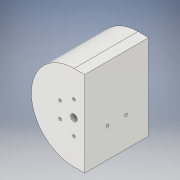
# Autodesk Inventor part: AA004
Saved by Autodesk Inventor 2017 SP1 (Build 210196100, 196)
## iProperties
Created: 2017-09-28
Part Number: AA004
Material: ABS Plastic
Document SubType Name: Modeling
Designer: Zach
Density: 1.06 g/cm^3
Appearance: CR White
Author: Zach
Autodesk Inventor part; units mm, degrees
ref_plane "YZ Plane" through (0, 0, 0) normal (1, 0, 0) x (0, 1, 0)
ref_plane "XZ Plane" through (0, 0, 0) normal (0, 1, 0) x (-1, 0, 0)
ref_plane "XY Plane" through (0, 0, 0) normal (0, 0, 1) x (1, 0, 0)
sketch "Sketch1" plane through (0, 0, 0) normal (0, 0, 1) x (1, 0, 0)
  circle A0 centre (0, 0) radius 80 construction
  line L0 (0, 80) -> (20, 80)
  line L1 (0, -80) -> (20, -80)
  line L2 (20, -80) -> (20, 80)
  arc A1 (0, 80) -> (0, -80) centre (0, 0) ccw
  circle A2 centre (0, 0) radius 6.15
  dimension "d0" = 160
  dimension "d1" = 20
  dimension "d3" = 12.3
  constraints: 6 end point, 4 point on circle, 3 centre point, 3 tangent, 2 coincident, 2 horizontal, 1 vertical alignment
  measures "d0" diameter of A0
  measures "d1" distance of L0.start L0.end
  measures "d3" diameter of A2
extrude "Extrusion1" add sketch "Sketch1" along normal blind 120
sketch "Sketch2" plane through (20, -80, 0) normal (1, 0, 0) x (0, 0, -1)
  line L0 (-120, 160) -> (-120, 0) projected
  line L1 (-120, 55.875) -> (0, 55.875) construction
  line L2 (0, 0) -> (0, 160) projected
  line L3 (-120, 0) -> (-120, 160) projected
  circle A0 centre (-42.5, 55.875) radius 2.5
  circle A1 centre (-77.5, 55.875) radius 2.5
  point P0 (0, 80)
  dimension "d6" = 24.125
  dimension "d7" = 5
  dimension "d8" = 5
  dimension "d9" = 42.5
  dimension "d10" = 35
  constraints: 5 point on line, 2 centre point, 2 end point, 1 horizontal
  measures "d6" distance from line of point (0, 80) L1
  measures "d7" diameter of A0
  measures "d8" diameter of A1
  measures "d9" distance from line of L2 A0.centre
  measures "d10" distance of A0.centre A1.centre
extrude "Extrusion2" cut sketch "Sketch2" against normal blind 35
sketch "Sketch3" plane through (0, 0, 120) normal (0, 0, 1) x (1, 0, 0)
  circle A0 centre (0, 30) radius 2.5
  circle A1 centre (-25.9808, 15) radius 2.5
  circle A2 centre (-25.9808, -15) radius 2.5
  circle A3 centre (0, -30) radius 2.5
  circle A4 centre (25.9808, -15) radius 2.5
  circle A5 centre (25.9808, 15) radius 2.5
  point P0 (0, 0)
  dimension "d14" = 5
  dimension "d15" = 30
  dimension "d18" = 360
  constraints: 6 centre point, 1 vertical alignment, 13 other
  measures "d14" diameter of A0
  measures "d15" distance of point (0, 0) A0.centre
extrude "Extrusion3" cut sketch "Sketch3" against normal through all
body "Solid1"
